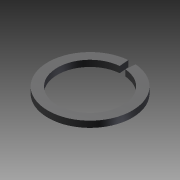
# Autodesk Inventor part: AT520
Saved by Autodesk Inventor 2011 SP1 (Build 150282100, 282)
## iProperties
Created: 2016-09-01
Part Number: AT520
Catalog Web Link: www.cadenas.de
Description: AT520 - Split Lockwasher-
Vendor: NKKSWITCHES
Document SubType Name: Modeling
Designer: psAdmin
Manufacturer: NKKSWITCHES
Mass: 0.0544144 g
Surface Area: 1.84863 cm^2
Volume: 0.0544144 cm^3
Density: 1 g/cm^3
Category: PARTsolutions
Company: NKKSWITCHES
Title: AT520
Author: Cadenas PARTsolutions
PSOL_IDENT_0: {$CADENAS_DATA\23d-libs\nkkswitches\rotary\hs_12_amp\parts\at520.prj},170 {VTYP=3D},{NB=AT520},{LINA=
PSOL_IDENT_1: AT520},{NN=AT520 - Split Lockwasher},{DATE=22.09.2015 06:04:15},{GEOMDATE=27.03.2009 08:37:00},{VERS
PSOL_IDENT_2: ION=},{LINEID=10},{LINESUBID=-1},{WBVAR=}  {NB=AT520},{LINA=AT520},{KT=DUMMY},{PN=AT520}
NN: AT520 - Split Lockwasher
NB: AT520
NBSYN: $PN.
LINA: AT520
PN: AT520
SUPPLIER: NKKSWITCHES
ARTICLENO: AT520
BOMINFO: AT520
CREATOR: CADENAS GmbH
Autodesk Inventor part; units mm, degrees
sketch "Sketch_1" plane through (0, 0, 0) normal (0, 1, 0) x (-1, 0, 0)
  arc A0 (0.5844, -6.6801) -> (-0.5844, -6.6801) centre (0, 0) ccw
  line L0 (-0.5844, -6.6801) -> (-0.4527, -5.1745)
  arc A1 (0.4527, -5.1745) -> (-0.4527, -5.1745) centre (0, 0) ccw
  line L1 (0.4527, -5.1745) -> (0.5844, -6.6801)
  constraints: 4 end point, 4 point on circle, 2 centre point
extrude "Extrusion1" add sketch "Sketch_1" along normal mid plane 0.9906
ref_plane "1_XY" through (0, 0, 0) normal (0, 1, 0) x (1, 0, 0)
ref_plane "1_YZ" through (0, 0, 0) normal (1, 0, 0) x (0, 0, -1)
ref_plane "1_ZX" through (0, 0, 0) normal (0, 0, -1) x (0, 1, 0)
body "Solid1"
